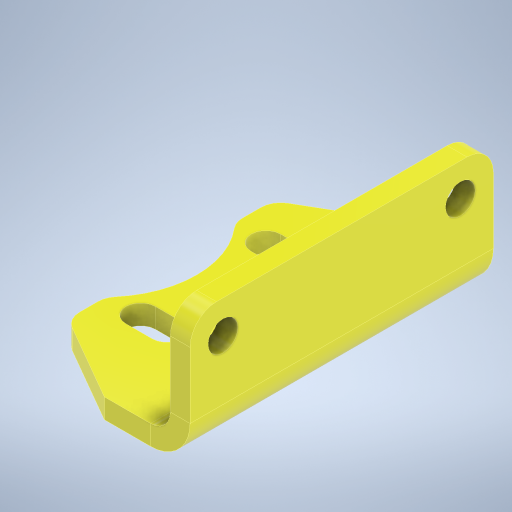
# Autodesk Inventor part: drzak_valce2
Saved by Autodesk Inventor 2024 (Build 280153000, 153)
## iProperties
Created: 2023-10-12
Part Number: drzak_valce2
Material: Železo, kujné
Document SubType Name: Sheet Metal
Designer: zak
Density: 7.15 g/cm^3
Sheet Metal Rule: Výchozí_mm
Appearance: Žlutá
Author: zak
Autodesk Inventor part; units mm, degrees
ref_plane "YZ Plane" through (0, 0, 0) normal (1, 0, 0) x (0, 1, 0)
ref_plane "XZ Plane" through (0, 0, 0) normal (0, 1, 0) x (-1, 0, 0)
ref_plane "XY Plane" through (0, 0, 0) normal (0, 0, 1) x (1, 0, 0)
sketch "Náčrt1" plane through (0, 0, 0) normal (0, 1, 0) x (-1, 0, 0)
  line L0 (0, 0) -> (26, 0)
  line L1 (13, -46) -> (0, -46)
  line L2 (0, -46) -> (0, 0)
  line L3 (26, -7.5056) -> (13, 0)
  line L4 (35.4765, -23) -> (0, -23) construction
  arc A0 (26, -13.202) -> (26, -32.798) centre (36, -23) ccw
  line L5 (26, -38.4944) -> (13, -46)
  line L6 (26, -7.5056) -> (26, -13.202)
  line L7 (26, -32.798) -> (26, -38.4944)
  point P0 (13, 0)
  dimension "d15" = -30
  dimension "d17" = 28
  dimension "d18" = 36
  dimension "d19" = 26
  dimension "d20" = 13
  dimension "d21" = 46
  dimension "d22" = 7.5056
  measures "d15" angle of L0 L3
  measures "d17" diameter of A0
  measures "d18" distance from line of A0.centre L2
  measures "d19" distance between parallel lines of L2 L6
  measures "d20" distance from line of L2 point (13, 0)
  measures "d21" distance between parallel lines of L1 L0
  measures "d22" distance from line of L0 L3.start
extrude "Deska1" add sketch "Náčrt1" along normal blind 3
sketch "Náčrt2" plane through (-3, 0, -46) normal (1, 0, 0) x (0, 1, 0)
  line L0 (0, 46) -> (0, 0)
  line L1 (0, 0) -> (20, 0)
  line L2 (20, 0) -> (20, 46)
  line L3 (20, 46) -> (0, 46)
  constraints: 6 end point, 1 horizontal, 1 perpendicular, 1 vertical
edge flange "Obruba1" height 20 angle 90 thickness 3 bend radius 3 thickness toward (1, 0, 0) relief tear relief width 3 relief depth 1.5 edges at (0, 3, -23) wall of the first edge with corners at (-3, 0, 0) (-3, 0, -46) (-3, 20, -46) (-3, 20, 0)
bend "Ohyb1"
corner "Roh1"
fillet "Zaoblení rohu1" radius 3 4 edges at (-26, 1.5, -7.5056) (-26, 1.5, -38.4944) (-26, 1.5, -13.202) (-26, 1.5, -32.798)
fillet "Zaoblení rohu2" radius 4 2 edges at (-1.5, 20, -46) (-1.5, 20, 0)
sketch "Náčrt3" plane through (-3, 6, -46) normal (-1, 0, 0) x (0, 0, 1)
  line L0 (42, 14) -> (4, 14) projected
  line L1 (23, 14) -> (23, 0) construction
  line L2 (46, 0) -> (0, 0) construction
  line L3 (0, -6) -> (46, -6) construction
  point P0 (41, 9)
  point P1 (5, 9)
  dimension "d25" = 36
  dimension "d26" = 15
  constraints: 2 end point, 2 midpoint, 1 symmetric about line
  measures "d25" distance of point (41, 9) point (5, 9)
  measures "d26" distance from line of L3 point (5, 9)
hole "Díra1" at (-3, 15, -5) at (-3, 15, -41) direction (1, 0, 0) diameter 4.5 end through all
sketch "Náčrt4" plane through (0, 3, 0) normal (0, 1, 0) x (1, 0, 0)
  line L0 (-21, 13.5) -> (-17, 13.5) construction
  line L1 (-21, 11.25) -> (-17, 11.25)
  line L2 (-17, 15.75) -> (-21, 15.75)
  arc A0 (-21, 15.75) -> (-21, 11.25) centre (-21, 13.5) ccw
  arc A1 (-17, 11.25) -> (-17, 15.75) centre (-17, 13.5) ccw
  arc A2 (-26, 13.202) -> (-26, 32.798) centre (-36, 23) ccw projected
  line L3 (-22, 23) -> (-6, 23) construction
  line L4 (-6, 0) -> (-6, 46) construction
  line L5 (-21, 32.5) -> (-17, 32.5) construction
  line L6 (-21, 34.75) -> (-17, 34.75)
  line L7 (-17, 30.25) -> (-21, 30.25)
  arc A3 (-21, 34.75) -> (-21, 30.25) centre (-21, 32.5) ccw
  arc A4 (-17, 30.25) -> (-17, 34.75) centre (-17, 32.5) ccw
  line L8 (-6, 0) -> (-13, 0) construction
  line L9 (-26, 9.2376) -> (-26, 13.202) construction
  point P0 (0, 0)
  point P1 (-19, 13.5)
  point P2 (-19, 32.5)
  point P3 (-19, 32.5)
  dimension "d36" = 4
  dimension "d37" = 4.5
  dimension "d40" = 19
  dimension "d41" = 5
  constraints: 18 end point, 9 point on circle, 7 symmetric about line, 4 centre point, 4 tangent, 3 midpoint, 3 parallel, 1 horizontal, 2 other
  measures "d36" distance of L0.start L0.end
  measures "d37" diameter of A1
  measures "d40" distance of point (-19, 32.5) point (-19, 13.5)
  measures "d41" distance from line of L9 L0.start
extrude "Vysunutí1" cut sketch "Náčrt4" against normal up to next
equation "\"d32\" = Tloušťka"
equation "\"d3\" = Tloušťka"
equation "\"d4\" = ŠířkaVýštipu"
equation "\"d5\" = HloubkaVýštipu"
equation "\"d6\" = MinimálníZbytek"
equation "\"d7\" = PřechodovýPoloměr"
equation "\"d10\" = PoloměrOhybu"
equation "\"d11\" = VelikostRohovéhoVýštipu"
equation "\"d12\" = VelikostMezery"
equation "\"d13\" = VelikostJacobihoPoloměru"
equation "\"PoloměrOhybu\" = Tloušťka"
equation "\"ŠířkaVýštipu\" = Tloušťka"
equation "\"HloubkaVýštipu\" = 0.5 * Tloušťka"
equation "\"VelikostRohovéhoVýštipu\" = 4 * Tloušťka"
equation "\"MinimálníZbytek\" = 2 * Tloušťka"
equation "\"PřechodovýPoloměr\" = PoloměrOhybu"
equation "\"VelikostJacobihoPoloměru\" = PoloměrOhybu"
equation "\"VelikostMezery\" = Tloušťka"
equation "\"Tloušťka\" = 3"
